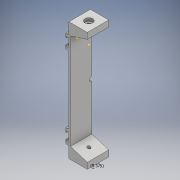
# Autodesk Inventor part: frontAxelHolder 8-14
Saved by Autodesk Inventor 2018 (Build 220112000, 112)
## iProperties
Created: 2019-08-08
Part Number: frontAxelHolder 8-14
Material: Generic
Document SubType Name: Modeling
Designer: Aditya Kendre
Density: 1 g/cm^3
Appearance: Default
Author: Aditya Kendre
## iProperties of the stored document rearAxelHolder 8-8_3DPrint.ipt
Created: 2019-08-08
Part Number: rearAxelHolder 8-8_3DPrint
Material: Generic
Document SubType Name: Modeling
Designer: Aditya Kendre
Density: 1 g/cm^3
Appearance: Default
Author: Aditya Kendre
Autodesk Inventor part; units mm, degrees
ref_plane "YZ Plane" through (0, 0, 0) normal (1, 0, 0) x (0, 1, 0)
ref_plane "XZ Plane" through (0, 0, 0) normal (0, 1, 0) x (-1, 0, 0)
ref_plane "XY Plane" through (0, 0, 0) normal (0, 0, 1) x (1, 0, 0)
sketch "Sketch1" plane through (0, 0, 0) normal (1, 0, 0) x (0, 1, 0)
  line L0 (0, 0) -> (24, 0)
  line L1 (24, 0) -> (24, -125)
  line L2 (24, -125) -> (0, -125)
  line L3 (0, -125) -> (0, 0)
  dimension "d0" = 24
  dimension "d1" = 125
  constraints: 8 end point, 2 parallel, 1 horizontal, 1 perpendicular
  measures "d0" distance of L1.end L2.end
  measures "d1" distance of L0.end L1.end
extrude "Extrusion1" add sketch "Sketch1" along normal blind 2
sketch "Sketch2" plane through (2, 0, 0) normal (1, 0, 0) x (0, 0, -1)
  line L0 (0, 24) -> (0, 0) projected
  line L1 (0, 0) -> (-15, 0)
  line L2 (-15, 0) -> (-15, 24)
  line L3 (-15, 24) -> (0, 24)
  line L4 (0, 24) -> (0, 0)
  line L5 (125, 0) -> (125, 24) projected
  line L6 (125, 24) -> (140, 24)
  line L7 (140, 24) -> (140, 0)
  line L8 (140, 0) -> (125, 0)
  line L9 (125, 0) -> (125, 24)
  dimension "d4" = 15
  dimension "d5" = 15
  constraints: 16 end point, 4 parallel, 2 horizontal, 2 perpendicular, 1 point on line
  measures "d4" distance of L2.end L3.end
  measures "d5" distance of L7.end L8.end
extrude "Extrusion2" add sketch "Sketch2" along normal blind 22 and the other way blind 2
sketch "Sketch3" plane through (24, 24, -140) normal (0, 0, -1) x (-1, 0, 0)
  line L0 (22, -24) -> (0, -24) construction
  line L1 (0, -24) -> (24, 0) construction
  line L2 (0, -24) -> (0, 0) construction
  line L3 (0, 0) -> (24, -24) construction
  circle A0 centre (12, -12) radius 11
  dimension "d10" = 22
  constraints: 4 end point, 1 centre point, 1 midpoint
  measures "d10" diameter of A0
extrude "Extrusion3" cut sketch "Sketch3" against normal blind 7.1
sketch "Sketch4" plane through (12, 12, -132.9) normal (0, 0, -1) x (-1, 0, 0)
  circle A0 centre (0, 0) radius 4.5
  point P0 (12, -12)
  dimension "d13" = 9
  constraints: 1 centre point
  measures "d13" diameter of A0
extrude "Extrusion4" cut sketch "Sketch4" against normal blind 155
sketch "Sketch5" plane through (0, 0, 15) normal (0, 0, 1) x (1, 0, 0)
  circle A0 centre (12, 12) radius 4.5 projected
  circle A1 centre (12, 12) radius 11
  point P0 (0, 0)
  dimension "d16" = 22
  constraints: 1 centre point, 1 coincident
  measures "d16" diameter of A1
extrude "Extrusion5" cut sketch "Sketch5" against normal blind 7.1
chamfer "Chamfer1" distance 7 angle 72.3 1 edges at (24, 12, -125)
sketch "Sketch6" plane through (24, 0, 0) normal (1, 0, 0) x (0, 0, -1)
  point P0 (0, 0)
chamfer "Chamfer2" distance 7 angle 72.3 1 edges at (24, 12, 0)
sketch "Sketch7" plane through (0, 0, 15) normal (0, -1, 0) x (1, 0, 0)
  line L0 (24, -155) -> (0, -155) projected
  line L1 (24, 0) -> (0, 0) projected
  line L2 (0, -155) -> (8, -155)
  line L3 (8, -155) -> (8, 0)
  line L4 (8, 0) -> (0, 0)
  line L5 (0, 0) -> (0, -155)
  point P0 (0, -15)
  dimension "d25" = 8
  constraints: 8 end point, 2 parallel, 1 horizontal, 1 perpendicular, 1 point on line
  measures "d25" distance of L4.end L3.end
sketch "Sketch8" plane through (24, 24, -140) normal (0, 0, -1) x (-1, 0, 0)
  point P0 (24, -24)
sketch "Sketch9" plane through (0, 24, -140) normal (0, 1, 0) x (1, 0, 0)
  point P0 (0, -140)
extrude "Extrusion6" add sketch "Sketch7" along normal blind 2
sketch "Sketch10" plane through (0, 24, -140) normal (0, 1, 0) x (1, 0, 0)
  line L0 (0, -155) -> (0, 0) projected
  line L1 (23, -155) -> (1, -155) projected
  line L2 (0, 0) -> (8, 0)
  line L3 (8, 0) -> (8, -155)
  line L4 (8, -155) -> (0, -155)
  line L5 (0, -155) -> (0, 0)
  point P0 (0, -140)
  dimension "d28" = 8
  constraints: 8 end point, 2 parallel, 1 horizontal, 1 perpendicular, 1 point on line
  measures "d28" distance of L3.end L4.end
extrude "Extrusion7" add sketch "Sketch10" along normal blind 2
sketch "Sketch11" plane through (24, 0, 7) normal (0, -1, 0) x (1, 0, 0)
  line L0 (0, 8) -> (-16, 8) projected
  line L1 (0, 8) -> (-16, 8)
  line L2 (-16, 8) -> (-16, -5.1062)
  line L3 (-16, 8) -> (-16, -147) projected
  line L4 (0, 0) -> (-16, -5.1063) projected
  line L5 (-16, -5.1063) -> (0, 0)
  line L6 (0, 0) -> (0, 8)
  line L7 (0, -147) -> (0, -139) projected
  line L8 (-16, -133.8937) -> (0, -139) projected
  line L9 (0, -139) -> (-16, -133.8937)
  line L10 (-16, -147) -> (-16, -133.8937) projected
  line L11 (-16, -133.8937) -> (-16, -147)
  line L12 (0, -147) -> (-16, -147) projected
  line L13 (-16, -147) -> (0, -147)
  line L14 (0, -147) -> (0, -139)
  point P0 (-24, -7)
  constraints: 16 end point, 5 collinear, 1 parallel, 1 perpendicular, 1 point on line
extrude "Extrusion8" add sketch "Sketch11" along normal blind 2
sketch "Sketch12" plane through (24, 24, -132) normal (0, 1, 0) x (1, 0, 0)
  line L0 (0, -139) -> (0, -147) projected
  line L1 (-16, -133.8937) -> (0, -139) projected
  line L2 (0, -139) -> (-16, -133.8937)
  line L3 (-16, -147) -> (-16, 8) projected
  line L4 (-16, -133.8937) -> (-16, -147)
  line L5 (0, -147) -> (-24, -147) projected
  line L6 (-16, -147) -> (0, -147)
  line L7 (0, -147) -> (0, -139)
  line L8 (0, 8) -> (-16, 8)
  line L9 (-24, 8) -> (0, 8) projected
  line L10 (-16, -5.1063) -> (-21.9339, -7) projected
  line L11 (-16, 8) -> (-16, -5.1063)
  line L12 (0, 8) -> (0, 0) projected
  line L13 (-16, -5.1063) -> (0, 0)
  line L14 (0, 0) -> (0, 8)
  point P0 (-24, -132)
  constraints: 16 end point, 3 perpendicular, 3 point on line, 2 collinear, 1 vertical
extrude "Extrusion9" add sketch "Sketch12" along normal blind 2
sketch "Sketch13" plane through (24, 0, 0) normal (1, 0, 0) x (0, 0, -1)
  point P0 (0, 0)
sketch "Sketch14" plane through (24, 0, 0) normal (1, 0, 0) x (0, 0, -1)
  point P0 (0, 0)
sketch "Sketch15" plane through (2, 0, 0) normal (1, 0, 0) x (0, 0, -1)
  line L0 (132, 26) -> (132, -2) construction
  line L1 (132, 12) -> (132, 6.5) construction
  line L2 (132, 6.5) -> (132, 17.5) construction
  line L3 (-7, -2) -> (-7, 26) projected
  line L4 (132, 6.5) -> (-7, 6.5)
  line L5 (-7, 6.5) -> (-7, 4.5)
  line L6 (-7, 4.5) -> (132, 4.5)
  line L7 (132, 4.5) -> (132, 6.5)
  line L8 (132, 17.5) -> (-7, 17.5)
  line L9 (-7, 17.5) -> (-7, 19.5)
  line L10 (-7, 19.5) -> (132, 19.5)
  line L11 (132, 19.5) -> (132, 17.5)
  point P0 (0, 0)
  dimension "d35" = 5.5
  dimension "d36" = 11
  dimension "d37" = 2
  dimension "d38" = 2
  constraints: 20 end point, 4 parallel, 4 point on line, 2 horizontal, 2 perpendicular, 1 midpoint
  measures "d35" distance of L1.start L1.end
  measures "d36" distance of L1.end L2.end
  measures "d37" distance of L5.end L4.end
  measures "d38" distance of L8.end L9.end
extrude "Extrusion10" add sketch "Sketch15" along normal blind 7
sketch "Sketch16" plane through (8, 0, 1.8937) normal (1, 0, 0) x (0, 0, -1)
  point P0 (1.8937, 0)
sketch "Sketch17" plane through (0, -2, 15) normal (0, -1, 0) x (1, 0, 0)
  line L0 (24, 0) -> (24, -8) projected
  line L1 (0, -155) -> (0, 0) projected
  line L2 (2.0661, -140) -> (2, -140) projected
  line L3 (8, -141.8937) -> (8, -13.1063) projected
  line L4 (8, -141.8937) -> (8, -13.1063)
  line L5 (8, -13.1063) -> (2.0661, -15) projected
  line L6 (2, -15) -> (8, -13.1063)
  line L7 (8, -141.8937) -> (8, -13.1063) projected
  line L8 (8, -13.1063) -> (8, -141.8937)
  line L9 (24, -147) -> (8, -141.8937) construction
  line L10 (2.0661, -140) -> (8, -141.8937) construction
  line L11 (8, -141.8937) -> (2.0661, -140) construction
  line L12 (8, -141.8937) -> (2, -140)
  line L13 (2, -140) -> (2, -15)
  line L14 (0, 0) -> (0, -155) projected
  point P0 (9, -12.7871)
  constraints: 14 end point, 3 collinear, 1 parallel
extrude "Extrusion11" cut sketch "Sketch17" against normal blind 2
fillet "Fillet1" radius 2 1 edges at (2, 4.5, -62.5)
fillet "Fillet2" radius 2 1 edges at (2, 19.5, -62.5)
sketch "Sketch18" plane through (2, 0, 0) normal (1, 0, 0) x (0, 0, -1)
  line L0 (0, 2.5) -> (0, 0) projected
  line L1 (0, 2.5) -> (125, 2.5)
  line L2 (125, 2.5) -> (125, -35.5)
  line L3 (125, -35.5) -> (0, -35.5)
  line L4 (0, -35.5) -> (0, 2.5)
  dimension "d46" = 38
  constraints: 8 end point, 2 parallel, 1 horizontal, 1 perpendicular
  measures "d46" distance of L1.end L2.end
extrude "Extrusion12" add sketch "Sketch18" against normal blind 2
sketch "Sketch19" plane through (2, 0, 0) normal (1, 0, 0) x (0, 0, -1)
  line L0 (125, -35.5) -> (0, -35.5) construction
  line L1 (62.5, -35.5) -> (62.5, 0) construction
  circle A0 centre (62.5, -17.75) radius 19 construction
  line L2 (125, -2) -> (125, -35.5) construction
  line L3 (62.5, -17.75) -> (81.5, -17.75) construction
  line L4 (81.5, -17.75) -> (103.25, -17.75) construction
  circle A1 centre (103.25, -17.75) radius 19 construction
  line L5 (62.5, -17.75) -> (21.75, -17.75) construction
  circle A2 centre (21.75, -17.75) radius 19 construction
  circle A3 centre (21.75, -17.75) radius 19
  circle A4 centre (62.5, -17.75) radius 19
  circle A5 centre (103.25, -17.75) radius 19
  circle A6 centre (103.25, -17.75) radius 20.375
  circle A7 centre (62.5, -17.75) radius 20.375
  circle A8 centre (21.75, -17.75) radius 20.375
  point P0 (0, 0)
  dimension "d49" = 38
  dimension "d51" = 43.5
  dimension "d52" = 21.75
  dimension "d53" = 38
  dimension "d54" = 40.75
  dimension "d55" = 38
  dimension "d56" = 40.75
  constraints: 8 centre point, 8 coincident, 8 end point, 3 horizontal, 2 concentric, 2 midpoint, 1 horizontal alignment, 1 vertical, 2 other
  measures "d51" distance from line of L2 L3.end
  measures "d52" distance of L3.end L4.end
  measures "d53" diameter of A1
  measures "d54" distance of L3.start L5.end
  measures "d55" diameter of A2
  measures "d56" diameter of A6
extrude "Extrusion13" add sketch "Sketch19" along normal blind 30
sketch "Sketch20" plane through (2, 0, 0) normal (-1, 0, 0) x (0, 0, 1)
  line L0 (-125, -35.5) -> (0, -35.5) projected
  line L1 (-125, -35.5) -> (0, -35.5)
  line L2 (0, -35.5) -> (0, -66.8086)
  line L3 (0, -66.8086) -> (-125, -66.8086)
  line L4 (-125, -66.8086) -> (-125, -35.5)
  point P0 (0, 0)
  constraints: 8 end point, 2 parallel, 1 horizontal, 1 perpendicular
extrude "Extrusion14" cut sketch "Sketch20" against normal blind 32
sketch "Sketch21" plane through (0, 0, 0) normal (-1, 0, 0) x (0, 0, 1)
  point P0 (0, 0)
sketch "Sketch22" plane through (0, 0, 0) normal (-1, 0, 0) x (0, 0, 1)
  line L0 (0, -35.5) -> (0, -2) projected
  line L1 (1.8937, 26) -> (-126.8937, 26) projected
  line L2 (0, -35.5) -> (-3, -35.5)
  line L3 (-3, -35.5) -> (-3, 26)
  line L4 (-3, 26) -> (0, 26)
  line L5 (0, 26) -> (0, -35.5)
  line L6 (-3, -35.5) -> (-15, -35.5) construction
  line L7 (-15, -35.5) -> (-15, 26) construction
  line L8 (-15, 26) -> (-3, 26) construction
  line L9 (-3, 26) -> (-3, -35.5) construction
  line L10 (-15, -35.5) -> (-18, -35.5)
  line L11 (-18, -35.5) -> (-18, 26)
  line L12 (-18, 26) -> (-15, 26)
  line L13 (-15, 26) -> (-15, -35.5)
  point P0 (0, 0)
  dimension "d61" = 3
  dimension "d62" = 12
  dimension "d63" = 3
  constraints: 24 end point, 6 parallel, 3 horizontal, 3 perpendicular, 3 point on line
  measures "d61" distance of L3.end L4.end
  measures "d62" distance of L7.end L8.end
  measures "d63" distance of L11.end L12.end
extrude "Extrusion15" add sketch "Sketch22" along normal blind 3.1
sketch "Sketch23" plane through (0, 0, 0) normal (-1, 0, 0) x (0, 0, 1)
  line L0 (1.8937, 26) -> (-126.8937, 26) projected
  line L1 (-125, -35.5) -> (-122, -35.5)
  line L2 (-122, -35.5) -> (-122, 26)
  line L3 (-122, 26) -> (-125, 26)
  line L4 (-125, 26) -> (-125, -35.5)
  line L5 (-125, -35.5) -> (-18, -35.5) construction
  line L6 (-122, 26) -> (-110, 26) construction
  line L7 (-110, 26) -> (-110, -35.5) construction
  line L8 (-110, -35.5) -> (-122, -35.5) construction
  line L9 (-122, -35.5) -> (-122, 26) construction
  line L10 (-140, 26) -> (-18, 26) construction
  line L11 (-110, -35.5) -> (-107, -35.5) construction
  line L12 (-107, -35.5) -> (-107, 26) construction
  line L13 (-107, 26) -> (-110, 26) construction
  line L14 (-110, 26) -> (-110, -35.5) construction
  line L15 (-110, 26) -> (-107, 26)
  line L16 (-107, 26) -> (-107, -35.5)
  line L17 (-107, -35.5) -> (-110, -35.5)
  line L18 (-110, -35.5) -> (-110, 26)
  point P0 (0, 0)
  dimension "d66" = 3
  dimension "d67" = 12
  dimension "d68" = 3
  constraints: 32 end point, 8 parallel, 4 horizontal, 4 perpendicular, 3 point on line
  measures "d66" distance of L3.end L2.end
  measures "d67" distance of L7.end L8.end
  measures "d68" distance of L13.end L12.end
extrude "Extrusion16" add sketch "Sketch23" along normal blind 3.1
sketch "Sketch24" plane through (0, 0, 0) normal (-1, 0, 0) x (0, 0, 1)
  point P0 (0, 0)
sketch "Sketch25" plane through (-3.1, 0, 0) normal (-1, 0, 0) x (0, 0, 1)
  point P0 (0, 0)
sketch "Sketch26" plane through (-3.1, 0, 0) normal (-1, 0, 0) x (0, 0, 1)
  line L0 (1.8937, 26) -> (-126.8937, 26) projected
  line L1 (-1.4573, 26) -> (-16.8386, 26)
  line L2 (-16.8386, 26) -> (-16.8386, 24)
  line L3 (-16.8386, 24) -> (-1.4573, 24)
  line L4 (-1.4573, 24) -> (-1.4573, 26)
  line L5 (-108.4459, 26) -> (-124.2367, 26)
  line L6 (-124.2367, 26) -> (-124.2367, 24)
  line L7 (-124.2367, 24) -> (-108.4459, 24)
  line L8 (-108.4459, 24) -> (-108.4459, 26)
  point P0 (0, 0)
  dimension "d71" = 2
  dimension "d72" = 2
  constraints: 16 end point, 4 parallel, 2 horizontal, 2 perpendicular, 2 point on line
  measures "d71" distance of L2.end L1.end
  measures "d72" distance of L6.end L5.end
extrude "Extrusion17" add sketch "Sketch26" against normal blind 3.6
sketch "Sketch27" plane through (-3.1, 0, 0) normal (-1, 0, 0) x (0, 0, 1)
  line L0 (-110, -35.5) -> (-107, -35.5) projected
  line L1 (-107, 26) -> (-125, 26) projected
  line L2 (-107, -35.5) -> (-112, -35.5)
  line L3 (-112, -35.5) -> (-112, 26)
  line L4 (-112, 26) -> (-107, 26)
  line L5 (-107, 26) -> (-107, -35.5)
  line L6 (-125, -35.5) -> (-113.2539, -35.5) projected
  line L7 (-125, -35.5) -> (-120, -35.5)
  line L8 (-120, -35.5) -> (-120, 26)
  line L9 (-120, 26) -> (-125, 26)
  line L10 (-125, 26) -> (-125, -35.5)
  line L11 (-11.7461, -35.5) -> (0, -35.5) projected
  line L12 (0, 26) -> (-18, 26) projected
  line L13 (0, -35.5) -> (-5, -35.5)
  line L14 (-5, -35.5) -> (-5, 26)
  line L15 (-5, 26) -> (0, 26)
  line L16 (0, 26) -> (0, -35.5)
  line L17 (-107, 26) -> (-18, 26) projected
  line L18 (-11.7461, -35.5) -> (-14.9723, -35.5) projected
  line L19 (-18, 26) -> (-13, 26)
  line L20 (-13, 26) -> (-13, -35.5)
  line L21 (-13, -35.5) -> (-18, -35.5)
  line L22 (-18, -35.5) -> (-18, 26)
  point P0 (0, 0)
  dimension "d75" = 5
  dimension "d76" = 5
  dimension "d77" = 5
  dimension "d78" = 5
  constraints: 32 end point, 8 parallel, 4 horizontal, 4 perpendicular, 4 point on line
  measures "d75" distance of L3.end L4.end
  measures "d76" distance of L9.end L8.end
  measures "d77" distance of L14.end L15.end
  measures "d78" distance of L20.end L21.end
extrude "Extrusion18" add sketch "Sketch27" along normal blind 1 contours L2 L3 L1 L5 L0 | L8 L6 L10 L1 | L14 L12 L16 L11 | L18 L21 L22 L12 L20
sketch "Sketch28" plane through (24, -2, -140) normal (0, 0, -1) x (-1, 0, 0)
  line L0 (0, 0) -> (0, 28) construction
  line L1 (0, 14) -> (0, 4.625) construction
  line L2 (21.9961, 4.625) -> (-8, 4.625) construction
  point P0 (24, 2)
  dimension "d81" = 9.375
  constraints: 2 end point, 1 midpoint, 1 point on line, 1 vertical
  measures "d81" distance of L1.start L1.end
fillet "Fillet3" radius 2 4 edges at (0, 12, -125) (0, -4.75, -107) (0, -4.75, -18) (0, 12, 0)
sketch "Sketch29" plane through (24, 0, 0) normal (1, 0, 0) x (0, 0, -1)
  line L0 (-15, -2) -> (-2, -2) projected
  line L1 (-15, -2) -> (143.5378, -2)
  line L2 (143.5378, -2) -> (143.5378, -41.4778)
  line L3 (143.5378, -41.4778) -> (-15, -41.4778)
  line L4 (-15, -41.4778) -> (-15, -2)
  point P0 (0, 0)
  constraints: 8 end point, 2 parallel, 1 horizontal, 1 perpendicular
extrude "Extrusion19" cut sketch "Sketch29" along normal mid plane 100
sketch "Sketch30" plane through (32, 0, 0) normal (1, 0, 0) x (0, 0, -1)
  line L0 (0, 26) -> (0, -2) projected
  line L1 (125, -2) -> (127, -2) projected
  line L2 (0, 2.5267) -> (125, 2.5267)
  line L3 (125, 2.5267) -> (125, -2)
  line L4 (125, -2) -> (0, -2)
  line L5 (0, -2) -> (0, 2.5267)
  line L6 (5, -2) -> (0, -2) projected
  line L7 (125, 3.0099) -> (125, 2.5) projected
  line L8 (0, -2) -> (125, -2)
  line L9 (125, -2) -> (125, 2.755)
  line L10 (125, 2.755) -> (0, 2.755)
  line L11 (0, 2.755) -> (0, -2)
  point P0 (0, 0)
  constraints: 16 end point, 4 parallel, 2 horizontal, 2 perpendicular, 1 midpoint, 1 point on line
extrude "Extrusion20" cut sketch "Sketch30" against normal blind 30
sketch "Sketch31" plane through (9, 0, 0) normal (1, 0, 0) x (0, 0, -1)
  point P0 (0, 0)
sketch "Sketch32" plane through (0, -2, 15) normal (0, -1, 0) x (1, 0, 0)
  line L0 (24, -8) -> (24, 0) projected
  line L1 (2, -15) -> (2.0661, -15) projected
  line L2 (24, -8) -> (2, -15)
  line L3 (2, -15) -> (2, -140)
  line L4 (0, -120) -> (0, -35) projected
  line L5 (2, -140) -> (24, -147.0211)
  line L6 (7.5, -141.7342) -> (16.5, -144.6064) projected
  line L7 (8, -13.1063) -> (24, -8) projected
  line L8 (24, -147.0211) -> (24, -8)
  point P0 (0, -15)
  constraints: 8 end point, 3 parallel
extrude "Extrusion21" cut sketch "Sketch32" against normal blind 30
sketch "Sketch33" plane through (0, -2, 15) normal (0, 0, 1) x (1, 0, 0)
  circle A0 centre (12, 14) radius 4.5 projected
  line L0 (24, 28) -> (24, 0) projected
  line L1 (0, 0) -> (0, 28) projected
  line L2 (24, 0) -> (0, 0)
  line L3 (0, 0) -> (0, 28)
  line L4 (0, 28) -> (24, 28)
  line L5 (24, 28) -> (24, 0)
  point P0 (0, 2)
  constraints: 8 end point, 2 parallel, 1 coincident, 1 horizontal, 1 perpendicular
extrude "Extrusion22" add sketch "Sketch33" against normal blind 8 contours A0 | L0 L2 L1 L4
sketch "Sketch34" plane through (0, 26, -140) normal (0, 1, 0) x (1, 0, 0)
  line L0 (2, -140) -> (24, -147) projected
  line L1 (2, -140) -> (2, -155)
  line L2 (24, -155) -> (0, -155) projected
  line L3 (2, -155) -> (24, -155)
  line L4 (24, -155) -> (24, -147) projected
  line L5 (24, -155) -> (24, -147)
  line L6 (24, -147) -> (2, -140)
  line L7 (0, 0) -> (24, 0) projected
  line L8 (24, -7.9789) -> (2.0097, -14.9969) projected
  line L9 (24, 0) -> (24, -7.9789)
  line L10 (24, -7.9789) -> (2.0097, -14.9969)
  line L11 (2.0097, -14.9969) -> (2, -0.0142)
  line L12 (2, -0.0142) -> (24, 0)
  line L13 (0, -13) -> (0, 0) projected
  line L14 (24, 0) -> (0, 0)
  line L15 (0, 0) -> (0, -7.5056)
  line L16 (0, -7.5056) -> (24, -7.5056)
  line L17 (24, -7.5056) -> (24, 0)
  point P0 (0, -140)
  constraints: 24 end point, 3 collinear, 2 parallel, 2 perpendicular, 2 point on line, 2 vertical, 1 horizontal
extrude "Extrusion23" add sketch "Sketch34" against normal blind 28
sketch "Sketch35" plane through (0, -2, 15) normal (0, 0, 1) x (1, 0, 0)
  line L0 (24, 28) -> (24, 0) construction
  line L1 (-3.1, 0) -> (0, 0) construction
  line L2 (24, 28) -> (0, 0) construction
  line L3 (0, 0) -> (24, 0) construction
  line L4 (0, 0) -> (24, 0) construction
  line L5 (0, 28) -> (0, 0) construction
  line L6 (24, 0) -> (0, 28) construction
  circle A0 centre (12, 14) radius 2
  point P0 (0, 2)
  dimension "d93" = 4
  constraints: 6 end point, 1 centre point, 1 collinear, 1 midpoint
  measures "d93" diameter of A0
extrude "Extrusion24" cut sketch "Sketch35" against normal blind 169
sketch "Sketch36" plane through (0, -2, 15) normal (0, 0, 1) x (1, 0, 0)
  circle A0 centre (12, 14) radius 2 projected
  circle A1 centre (12, 14) radius 5
  point P0 (0, 2)
  dimension "d96" = 10
  constraints: 1 centre point, 1 coincident
  measures "d96" diameter of A1
extrude "Extrusion25" cut sketch "Sketch36" against normal blind 4
sketch "Sketch37" plane through (24, -2, -140) normal (0, 0, -1) x (-1, 0, 0)
  circle A0 centre (12, 14) radius 2 projected
  circle A1 centre (12, 14) radius 5
  point P0 (24, 2)
  constraints: 1 centre point, 1 coincident
extrude "Extrusion26" cut sketch "Sketch37" against normal blind 4
sketch "Sketch38" plane through (2, 0, 0) normal (1, 0, 0) x (0, 0, -1)
  line L0 (105, 26) -> (20, 26) construction
  circle A0 centre (62.5, 26) radius 3.175 construction
  circle A1 centre (62.5, 26) radius 3.175
  point P0 (0, 0)
  dimension "d101" = 6.35
  constraints: 2 centre point, 1 coincident, 1 concentric, 1 midpoint
  measures "d101" diameter of A0
extrude "Extrusion27" cut sketch "Sketch38" against normal blind 40
sketch "Sketch39" plane through (0, 0, 0) normal (-1, 0, 0) x (0, 0, 1)
  line L0 (-65.675, 26) -> (-66.675, 26)
  line L1 (-105, 26) -> (-65.675, 26) projected
  line L2 (0, 26) -> (-59.325, 26) projected
  line L3 (-59.325, 26) -> (-58.325, 26)
  line L4 (-66.675, 26) -> (-58.325, 26) construction
  arc A0 (-66.675, 26) -> (-58.325, 26) centre (-62.5, 26.0125) ccw
  arc A1 (-65.675, 26) -> (-59.325, 26) centre (-62.5, 26) ccw
  point P0 (0, 0)
  dimension "d104" = 1
  dimension "d105" = 1
  constraints: 6 end point, 4 point on circle, 2 centre point, 2 point on line, 1 collinear
  measures "d104" distance of L0.start L0.end
  measures "d105" distance of L2.end L3.end
extrude "Extrusion28" add sketch "Sketch39" along normal blind 5
fillet "Fillet4" radius 2 1 edges at (0, 21.8375, -62.5)
body "Solid1"
